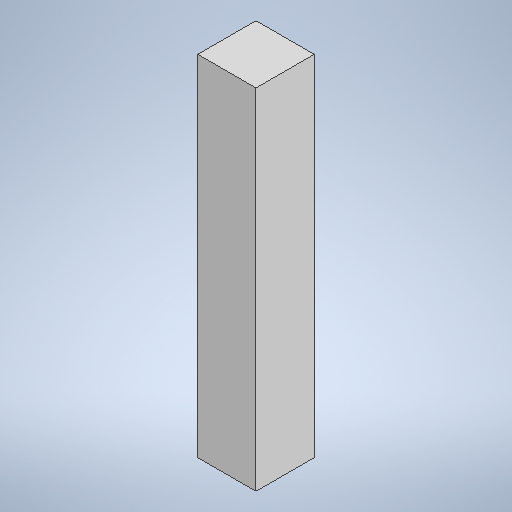
# Autodesk Inventor part: stand1
Saved by Autodesk Inventor 2025.2 (Build 292293000, 293)
## iProperties
Created: 2025-04-11
Part Number: stand1
Material: Generic
Document SubType Name: Modeling
Designer: joaki
Density: 1 g/cm^3
Appearance: Default
Author: joaki
Autodesk Inventor part; units mm, degrees
ref_plane "YZ Plane" through (0, 0, 0) normal (1, 0, 0) x (0, 1, 0)
ref_plane "XZ Plane" through (0, 0, 0) normal (0, 1, 0) x (-1, 0, 0)
ref_plane "XY Plane" through (0, 0, 0) normal (0, 0, 1) x (1, 0, 0)
sketch "Sketch1" plane through (0, 0, 0) normal (0, 1, 0) x (-1, 0, 0)
  line L0 (2.4215, 2.9174) -> (-3.5785, 2.9174)
  line L1 (-3.5785, 2.9174) -> (-3.5785, -3.0826)
  line L2 (-3.5785, -3.0826) -> (2.4215, -3.0826)
  line L3 (2.4215, -3.0826) -> (2.4215, 2.9174)
  point P0 (0, 0)
  dimension "d0" = 6
  dimension "d1" = 6
  constraints: 8 end point, 2 parallel, 1 horizontal, 1 perpendicular
  measures "d0" distance between parallel lines of L3 L1
  measures "d1" distance of L2.end L0.start
extrude "Extrusion1" add sketch "Sketch1" along normal blind 36
body "Solid1"
